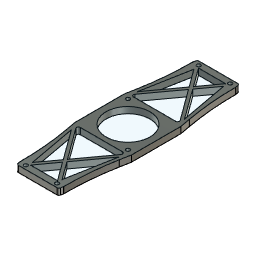
stepper_holding_bracket_printer v3 (Autodesk Fusion 360 design; units mm, degrees)
Autodesk Fusion 360 part; units mm, degrees
note: some values were not read from the file. Set by a fixed rule: which face or edge a step refers to.
sketch "Sketch1" plane through (0, 0, 0) normal (0, 0, 1) x (1, 0, 0)
  line L0 (-21.15, 21.15) -> (21.15, -21.15) construction
  line L1 (21.15, -21.15) -> (-21.15, -21.15)
  line L2 (-21.15, 21.15) -> (-19.0287, 19.0287) construction
  circle A0 centre (0, 0) radius 11
  line L3 (19.0287, 19.0287) -> (21.15, 16.9074)
  line L4 (21.15, 21.15) -> (19.0287, 19.0287) construction
  line L5 (-19.0287, -19.0287) -> (-16.9074, -21.15)
  line L6 (-19.0287, -19.0287) -> (-15.4931, -15.4931) construction
  line L7 (19.0287, 19.0287) -> (16.9074, 21.15)
  line L8 (-19.0287, 19.0287) -> (-21.15, 16.9074)
  line L9 (-19.0287, 19.0287) -> (-16.9074, 21.15)
  line L10 (-21.15, -21.15) -> (-21.15, 21.15)
  line L11 (19.0287, -19.0287) -> (16.9074, -21.15)
  line L12 (-19.0287, 19.0287) -> (-15.4931, 15.4931) construction
  line L13 (-19.0287, -19.0287) -> (-21.15, -16.9074)
  line L14 (21.15, 21.15) -> (-21.15, -21.15) construction
  line L15 (-21.15, -21.15) -> (-19.0287, -19.0287) construction
  line L16 (19.0287, -19.0287) -> (15.4931, -15.4931) construction
  line L17 (21.15, -21.15) -> (19.0287, -19.0287) construction
  line L18 (19.0287, -19.0287) -> (21.15, -16.9074)
  line L19 (19.0287, 19.0287) -> (15.4931, 15.4931) construction
  line L20 (21.15, 21.15) -> (21.15, -21.15)
  line L21 (-21.15, 21.15) -> (21.15, 21.15)
  circle A1 centre (0, 0) radius 2.5
  line L22 (22.5, 75) -> (-14.9629, 75)
  line L23 (-22.5, 75) -> (-22.5, -75)
  line L24 (-22.5, -75) -> (22.5, -75)
  line L25 (22.5, -75) -> (22.5, 75)
  line L26 (22.5, 75) -> (-22.5, -75) construction
  line L27 (-22.5, 75) -> (22.5, -75) construction
  line L28 (-22.5, 69) -> (22.5, 69) construction
  circle A2 centre (-12.5, 69) radius 1.5
  line L29 (-22.5, 0) -> (22.5, 0) construction
  line L30 (0, 75) -> (0, -75) construction
  circle A3 centre (12.5, 69) radius 1.5
  line L31 (-15.7993, 67) -> (22.5, 67)
  line L32 (-12.5559, 67.501) -> (-21.15, 21.15)
  line L33 (-22.5, 19.721) -> (-13.5598, 67.9385)
  line L34 (-21.15, 21.15) -> (-19.8211, 21.15) construction
  line L35 (-19.8211, 21.15) -> (-11.025, 68.7273)
  line L36 (21.15, 21.15) -> (-12.5559, 67.501)
  line L37 (22.5, 21.2586) -> (-11.443, 67.9357)
  line L38 (21.15, 21.15) -> (19.8211, 21.15) construction
  line L39 (-17.2787, 68.7475) -> (-16.4423, 73.7475)
  line L40 (19.8211, 21.15) -> (-13.7338, 67)
  arc A4 (-17.2787, 68.7475) -> (-15.7993, 67) centre (-15.7993, 68.5) ccw
  arc A5 (-14.9629, 75) -> (-16.4423, 73.7475) centre (-14.9629, 73.5) ccw
  line L41 (22.5, 19.721) -> (13.5598, 67.9385)
  line L42 (19.8211, 21.15) -> (11.025, 68.7273)
  line L43 (-19.8211, 21.15) -> (13.7338, 67)
  line L44 (-22.5, 21.2586) -> (11.443, 67.9357)
  arc A6 (15.7993, 67) -> (17.2787, 68.7475) centre (15.7993, 68.5) ccw
  line L45 (17.2787, 68.7475) -> (16.4423, 73.7475)
  arc A7 (16.4423, 73.7475) -> (14.9629, 75) centre (14.9629, 73.5) ccw
  line L46 (-22.5, -19.721) -> (-13.5598, -67.9385)
  line L47 (-19.8211, -21.15) -> (-11.025, -68.7273)
  line L48 (19.8211, -21.15) -> (-13.7338, -67)
  line L49 (22.5, -21.2586) -> (-11.443, -67.9357)
  line L50 (-22.5, -21.2586) -> (11.443, -67.9357)
  line L51 (-19.8211, -21.15) -> (13.7338, -67)
  line L52 (19.8211, -21.15) -> (11.025, -68.7273)
  line L53 (22.5, -19.721) -> (13.5598, -67.9385)
  circle A8 centre (12.5, -69) radius 1.5
  circle A9 centre (-12.5, -69) radius 1.5
  arc A10 (-15.7993, -67) -> (-17.2787, -68.7475) centre (-15.7993, -68.5) ccw
  line L54 (-17.2787, -68.7475) -> (-16.4423, -73.7475)
  arc A11 (-16.4423, -73.7475) -> (-14.9629, -75) centre (-14.9629, -73.5) ccw
  arc A12 (14.9629, -75) -> (16.4423, -73.7475) centre (14.9629, -73.5) ccw
  line L55 (17.2787, -68.7475) -> (16.4423, -73.7475)
  arc A13 (17.2787, -68.7475) -> (15.7993, -67) centre (15.7993, -68.5) ccw
  line L56 (-15.7993, -67) -> (22.5, -67)
  line L57 (0, 0) -> (-17.5716, 17.5716) construction
  line L58 (0, 0) -> (17.5716, -17.5716) construction
  circle A14 centre (17.5716, -17.5716) radius 1.5
  circle A15 centre (-17.5716, 17.5716) radius 1.5
  dimension "d1" = 42.3
  dimension "d2" = 42.3
  dimension "d3" = 3
  dimension "d4" = 3
  dimension "d5" = 3
  dimension "d6" = 3
  dimension "d15" = 5
  dimension "d16" = 22
  dimension "d17" = 45
  dimension "d18" = 150
  dimension "d19" = 6
  dimension "d20" = 3
  dimension "d21" = 10
  dimension "d22" = 8
  dimension "d23" = 1.3289
  dimension "d24" = 1.3289
  dimension "d25" = 1.5
  dimension "d26" = 1.5
  dimension "d50" = 24.85
  dimension "d51" = 24.85
  dimension "d52" = 3
  dimension "d53" = 3
  constraint horizontal L21
  constraint vertical L20
  constraint horizontal L1
  constraint vertical L10
  constraint coincident L5.start L14
  constraint perpendicular L2 L15
  constraint coincident L3.start L14
  constraint coincident L11.start L0
  constraint coincident L11.end L1
  constraint perpendicular L0 L11
  constraint coincident L18.end L20
  constraint perpendicular L0 L18
  constraint coincident L5.end L1
  constraint perpendicular L5 L15
  constraint coincident L13.end L10
  constraint perpendicular L13 L14
  constraint coincident L8.end L10
  constraint perpendicular L0 L8
  constraint coincident L9.end L21
  constraint perpendicular L0 L9
  constraint coincident L3.end L20
  constraint perpendicular L3 L14
  constraint coincident L7.end L21
  constraint perpendicular L4 L7
  constraint coincident L19.end L14
  constraint coincident L12.end L0
  constraint coincident L6.end L14
  constraint coincident L16.end L0
  constraint midpoint A0.centre L0
  constraint concentric A0 A1
  constraint horizontal L22
  constraint perpendicular L22 L23
  constraint parallel L22 L24
  constraint parallel L23 L25
  constraint coincident L26 A0.centre
  constraint coincident L27 A0.centre
  constraint coincident A0.centre A1.centre
  constraint coincident L23 L28.start
  constraint coincident L25 L28.end
  constraint perpendicular L25 L28
  constraint coincident L28 A2.centre
  constraint midpoint L23 L29.start
  constraint midpoint L25 L29.end
  constraint midpoint L24 L30.end
  constraint symmetric A2 L30 A3
  constraint coincident L25 L31.end
  constraint perpendicular L25 L31
  constraint coincident A2 L32.start
  constraint coincident L23 L33.start
  constraint coincident A2 L33.end
  constraint parallel L32 L33
  constraint coincident L21 L34.end
  constraint coincident A2 L35.end
  constraint tangent A2 L35
  constraint coincident L25 L37.start
  constraint coincident A2 L37.end
  constraint parallel L36 L37
  constraint coincident L21 L38.end
  constraint coincident L33 L40.end
  constraint tangent L39 A4
  constraint tangent L31 A4
  constraint coincident L22 L30.start
  constraint coincident L23.start L22
  constraint tangent L39 A5
  constraint tangent L22 A5
  constraint symmetric L30 L33.start L41.start
  constraint symmetric L30 L33.end L41.end
  constraint symmetric L30 L34.end L38.end
  constraint symmetric L30 L35.end L42.end
  constraint symmetric L30 L37.start L44.start
  constraint symmetric L30 L37.end L44.end
  constraint symmetric L30 L38.end L34.end
  constraint symmetric L30 L40.end L43.end
  constraint symmetric L30 L39.start A6.end
  constraint symmetric L30 L31.start A6.start
  constraint symmetric L30 A4 A6
  constraint symmetric L30 L39.end L45.end
  constraint symmetric L30 L22.end A7.end
  constraint symmetric L30 A5 A7
  constraint symmetric A2 L29 A9
  constraint symmetric L29 A3 A8
  constraint symmetric L29 L31.end L56.end
  constraint symmetric L29 L33.start L46.start
  constraint symmetric L29 L33.end L46.end
  constraint symmetric L29 L34.end L47.start
  constraint symmetric L29 L35.end L47.end
  constraint symmetric L29 L37.start L49.start
  constraint symmetric L29 L37.end L49.end
  constraint symmetric L29 L38.end L48.start
  constraint symmetric L29 L40.end L48.end
  constraint symmetric L29 L39.start A10.end
  constraint symmetric L29 L31.start A10.start
  constraint symmetric L29 A4 A10
  constraint symmetric L29 L39.end L54.end
  constraint symmetric L29 L22.end A11.end
  constraint symmetric L29 A5 A11
  constraint symmetric L29 L41.start L53.start
  constraint symmetric L29 L41.end L53.end
  constraint symmetric L29 L42.end L52.end
  constraint symmetric L29 L43.end L51.end
  constraint symmetric L29 L44.start L50.start
  constraint symmetric L29 L44.end L50.end
  constraint symmetric L29 A6.end L55.start
  constraint symmetric L29 A6.start A13.end
  constraint symmetric L29 A6 A13
  constraint symmetric L29 L45.end A12.end
  constraint symmetric L29 A7.end A12.start
  constraint symmetric L29 A7 A12
  constraint coincident L31 L40.end
  constraint parallel L0 L57
  constraint coincident L16 L58.end
  constraint coincident L58.end A14.centre
  constraint coincident L57.end A15.centre
  measures "d1" distance of L1.end L0.start
  measures "d2" distance of L0.start L4.start
  measures "d3" distance of L1.end L5.start
  measures "d4" distance of L0.start L2.end
  measures "d5" distance of L4.start L3.start
  measures "d6" distance of L11.start L0.end
  measures "d15" diameter of A1
  measures "d16" diameter of A0
  measures "d17" distance of L23.end L24.end
  measures "d18" distance of L23.start L23.end
  measures "d19" distance of L22 L28
  measures "d20" diameter of A2
  measures "d21" distance of L23 A2.centre
  measures "d22" distance of L22 L31
  measures "d23" distance of L0.start L34.end
  measures "d24" distance of L4.start L38.end
  measures "d25" radius of A4
  measures "d26" radius of A5
  measures "d50" distance of A0.centre L57.end
  measures "d51" distance of A0.centre L58.end
  measures "d52" diameter of A14
  measures "d53" diameter of A15
extrude "Extrude1" add sketch "Sketch1" along normal blind 5 contours L1 L20 L25 L36 L37 L41 L42 L49 L52 L53 | L1 L11 L18 L20 | L48 L49 L51 L52 | L1 L3 L5 L7 L8 L9 L10 L11 L13 L18 L20 L21 | L48 L49 L50 L51 | L47 L48 L50 L51 | L49 L51 L52 L53 | L3 L7 L20 L21 | L1 L5 L10 L13 | L47 L48 L49 L50 L56 | L1 L10 L23 L32 L33 L44 L46 L47 L50 | L49 L50 L51 L52 L56 | L51 L52 L56 | L21 L36 L42 | L46 L47 L48 L50 | L47 L48 L56 | L24 L46 L47 L49 L50 L52 L53 A8 A9 A10 L54 A11 A12 L55 A13 L56 | L50 L52 L53 A8 L56 | L50 L52 L56 | L36 L40 L42 L43 | L36 L37 L42 L43 | L47 L49 L56 | L46 L47 L49 A9 L56 | L50 L52 A8 | L8 L9 L10 L21 | L35 L40 L43 L44 | L36 L40 L43 L44 | L36 L37 L43 L44 | L37 L41 L42 L43 | L47 L49 A9 | L21 L32 L35 L44 | L35 L36 L40 L44 | L31 L35 L36 L37 L44 | L31 L37 L42 L43 L44 | L31 L42 L43 | L22 A2 A3 L31 L33 L35 L37 L39 A4 A5 L41 L42 L44 A6 L45 A7 | A3 L31 L41 L42 L44 | L32 L35 L40 L44 | L31 L32 L35 L36 L40 | L31 L35 L36 | L31 L42 L44 | L32 L33 L40 L44 | L31 L32 L40 | L31 L35 L37 | A2 L31 L35 L36 L37 | L31 L32 L36 | A3 L42 L44 | A2 L31 L32 L33 | A2 L35 L37 | A14 | A15
fillet "Fillet1" radius 1.5 4 edges at (19.8211, 21.15, 2.5) (-19.8211, 21.15, 2.5) (19.8211, -21.15, 2.5) (-19.8211, -21.15, 2.5)
fillet "Fillet2" radius 219.5 4 edges at (-13.7338, 67, 2.5) (13.7338, 67, 2.5) (-13.7338, -67, 2.5) (13.7338, -67, 2.5)
sketch "Sketch2" plane through (0, 0, 5) normal (0, 0, 1) x (-1, 0, 0)
  line L0 (-11.8262, -64.3935) -> (-18.8809, -26.2354)
  line L1 (-18.8809, -26.2354) -> (-1.4466, -50.2105)
  line L2 (-1.4466, -50.2105) -> (-11.8262, -64.3935)
  circle A0 centre (-12.5, -69) radius 1.5
  line L3 (18.8809, 26.2354) -> (1.4466, 50.2105)
  line L4 (1.4466, 50.2105) -> (11.8262, 64.3935)
  line L5 (11.8262, 64.3935) -> (18.8809, 26.2354)
  line L6 (10.7626, 67) -> (0, 52.1997)
  line L7 (0, 52.1997) -> (-10.7626, 67)
  line L8 (-10.7626, 67) -> (10.7626, 67)
  circle A1 centre (12.5, 69) radius 1.5
  circle A2 centre (-12.5, 69) radius 1.5
  line L9 (0, -48.2339) -> (-18.075, -23.5359)
  arc A3 (-16.8646, -21.15) -> (-18.075, -23.5359) centre (-16.8646, -22.65) ccw
  line L10 (-16.8646, -21.15) -> (16.8646, -21.15)
  arc A4 (18.075, -23.5359) -> (16.8646, -21.15) centre (16.8646, -22.65) ccw
  line L11 (18.075, -23.5359) -> (0, -48.2339)
  circle A5 centre (12.5, -69) radius 1.5
  line L12 (16.8646, 21.15) -> (-16.8646, 21.15)
  arc A6 (-18.075, 23.5359) -> (-16.8646, 21.15) centre (-16.8646, 22.65) ccw
  line L13 (-18.075, 23.5359) -> (0, 48.2339)
  line L14 (0, 48.2339) -> (18.075, 23.5359)
  arc A7 (16.8646, 21.15) -> (18.075, 23.5359) centre (16.8646, 22.65) ccw
  line L15 (-10.7626, -67) -> (0, -52.1997)
  line L16 (0, -52.1997) -> (10.7626, -67)
  line L17 (10.7626, -67) -> (-10.7626, -67)
  line L18 (11.8262, -64.3935) -> (1.4466, -50.2105)
  line L19 (1.4466, -50.2105) -> (18.8809, -26.2354)
  line L20 (18.8809, -26.2354) -> (11.8262, -64.3935)
  circle A8 centre (0, 0) radius 11
  line L21 (-1.4466, 50.2105) -> (-18.8809, 26.2354)
  line L22 (-18.8809, 26.2354) -> (-11.8262, 64.3935)
  line L23 (-11.8262, 64.3935) -> (-1.4466, 50.2105)
  line L24 (17.2787, 68.7475) -> (16.4423, 73.7475)
  arc A9 (16.4423, 73.7475) -> (14.9629, 75) centre (14.9629, 73.5) ccw
  line L25 (14.9629, 75) -> (-14.9629, 75)
  arc A10 (-14.9629, 75) -> (-16.4423, 73.7475) centre (-14.9629, 73.5) ccw
  line L26 (-16.4423, 73.7475) -> (-17.2787, 68.7475)
  arc A11 (-17.2787, 68.7475) -> (-17.2992, 68.4963) centre (-15.7993, 68.5) ccw
  arc A12 (-20.977, 27.9349) -> (-17.2992, 68.4963) centre (-236.7986, 67.9512) ccw
  line L27 (-20.977, 27.9349) -> (-22.5, 19.721)
  line L28 (-22.5, 19.721) -> (-22.5, -19.721)
  line L29 (-22.5, -19.721) -> (-20.977, -27.9349)
  arc A13 (-17.2992, -68.4963) -> (-20.977, -27.9349) centre (-236.7986, -67.9512) ccw
  arc A14 (-17.2992, -68.4963) -> (-17.2787, -68.7475) centre (-15.7993, -68.5) ccw
  line L30 (-17.2787, -68.7475) -> (-16.4423, -73.7475)
  arc A15 (-16.4423, -73.7475) -> (-14.9629, -75) centre (-14.9629, -73.5) ccw
  line L31 (-14.9629, -75) -> (14.9629, -75)
  arc A16 (14.9629, -75) -> (16.4423, -73.7475) centre (14.9629, -73.5) ccw
  line L32 (16.4423, -73.7475) -> (17.2787, -68.7475)
  arc A17 (17.2787, -68.7475) -> (17.2992, -68.4963) centre (15.7993, -68.5) ccw
  arc A18 (20.977, -27.9349) -> (17.2992, -68.4963) centre (236.7986, -67.9512) ccw
  line L33 (20.977, -27.9349) -> (22.5, -19.721)
  line L34 (22.5, -19.721) -> (22.5, 19.721)
  line L35 (22.5, 19.721) -> (20.977, 27.9349)
  arc A19 (17.2992, 68.4963) -> (20.977, 27.9349) centre (236.7986, 67.9512) ccw
  arc A20 (17.2992, 68.4963) -> (17.2787, 68.7475) centre (15.7993, 68.5) ccw
  circle A21 centre (-15.4931, 15.4931) radius 3.5
  line L36 (-22.5, 0) -> (22.5, 0) construction
  line L37 (0, 0) -> (0, 75) construction
  circle A22 centre (15.4931, 15.4931) radius 3.5
  line L38 (-15.4931, 15.4931) -> (-11.9931, 15.4931) construction
  circle A23 centre (0, 142.5886) radius 124.5363 construction
  circle A24 centre (0, 142.5886) radius 131.5363 construction
  circle A25 centre (0, 0) radius 13.5
  arc A26 (-13.268, 2.4919) -> (-17.4643, 12.601) centre (-23.0962, 4.3377) ccw
  arc A27 (-12.601, 17.4643) -> (-2.4919, 13.268) centre (-4.3377, 23.0962) ccw
  arc A28 (17.4643, 12.601) -> (13.268, 2.4919) centre (23.0962, 4.3377) ccw
  arc A29 (2.4919, 13.268) -> (12.601, 17.4643) centre (4.3377, 23.0962) ccw
  arc A30 (-17.4643, -12.601) -> (-13.268, -2.4919) centre (-23.0962, -4.3377) ccw
  arc A31 (-2.4919, -13.268) -> (-12.601, -17.4643) centre (-4.3377, -23.0962) ccw
  circle A32 centre (-15.4931, -15.4931) radius 3.5
  arc A33 (12.601, -17.4643) -> (2.4919, -13.268) centre (4.3377, -23.0962) ccw
  arc A34 (13.268, -2.4919) -> (17.4643, -12.601) centre (23.0962, -4.3377) ccw
  circle A35 centre (15.4931, -15.4931) radius 3.5
  line L39 (-15.4931, 15.4931) -> (-15.4931, 18.9931) construction
  line L40 (-15.4931, 18.9931) -> (15.4931, 18.9931)
  line L41 (-18.9931, 15.4931) -> (-18.9931, -15.4931)
  line L42 (-15.4931, -18.9931) -> (15.4931, -18.9931)
  line L43 (18.9931, -15.4931) -> (18.9931, 15.4931)
  line L44 (13.105, 4.7569) -> (13.105, -4.7569)
  line L45 (-13.105, 4.7569) -> (-13.105, -4.7569)
  line L46 (4.7605, -0.0581) -> (-4.7533, -0.0581)
  line L47 (0, 0) -> (0, -13.105) construction
  line L48 (0, -13.105) -> (4.3174, -13.0962) construction
  line L49 (4.3174, -13.0962) -> (-4.3377, -13.0962)
  line L50 (4.3174, 13.0962) -> (-4.3377, 13.0962)
  arc A36 (16.9784, -12.248) -> (18.9931, -11.2592) centre (17.7431, -11.2592) ccw
  arc A37 (11.2592, -18.9931) -> (12.248, -16.9784) centre (11.2592, -17.7431) ccw
  arc A38 (-12.248, -16.9784) -> (-11.2592, -18.9931) centre (-11.2592, -17.7431) ccw
  arc A39 (-18.9931, -11.2592) -> (-16.9784, -12.248) centre (-17.7431, -11.2592) ccw
  arc A40 (18.9931, 11.2592) -> (16.9784, 12.248) centre (17.7431, 11.2592) ccw
  arc A41 (12.248, 16.9784) -> (11.2592, 18.9931) centre (11.2592, 17.7431) ccw
  arc A42 (-11.2592, 18.9931) -> (-12.248, 16.9784) centre (-11.2592, 17.7431) ccw
  arc A43 (-16.9784, 12.248) -> (-18.9931, 11.2592) centre (-17.7431, 11.2592) ccw
  dimension "d33" = 7
  dimension "d36" = 7
  dimension "d37" = 27
  dimension "d38" = 20
  dimension "d39" = 20
  dimension "d40" = 13.105
  dimension "d43" = 2.5
  dimension "d44" = 2.5
  constraint midpoint L28 L36.start
  constraint midpoint L34 L36.end
  constraint coincident A8.centre L37.start
  constraint midpoint L25 L37.end
  constraint symmetric A21 L37 A22
  constraint horizontal L38
  constraint tangent A21 A23
  constraint tangent A22 A23
  constraint tangent A21 A26
  constraint tangent A25 A26
  constraint tangent A25 A27
  constraint tangent A21 A27
  constraint coincident A25 A26.start
  constraint coincident A21 A26.end
  constraint coincident A25 A27.end
  constraint coincident A21 A27.start
  constraint symmetric L37 A26.start A28.end
  constraint symmetric L37 A26.end A28.start
  constraint symmetric L37 A26 A28
  constraint symmetric L37 A27.end A29.start
  constraint symmetric L37 A27 A29
  constraint symmetric L37 A27.start A29.end
  constraint symmetric A21 L36 A32
  constraint symmetric L36 A22 A35
  constraint symmetric L36 A26.start A30.end
  constraint symmetric L36 A26.end A30.start
  constraint symmetric L36 A26 A30
  constraint symmetric L36 A27.end A31.start
  constraint symmetric L36 A27 A31
  constraint symmetric L36 A27.start A31.end
  constraint symmetric L36 A28.end A34.start
  constraint symmetric L36 A28.start A34.end
  constraint symmetric L36 A28 A34
  constraint symmetric L36 A29.end A33.start
  constraint symmetric L36 A29.start A33.end
  constraint symmetric L36 A29 A33
  constraint coincident A21 L39.end
  constraint perpendicular L38 L39
  constraint coincident A22 L40.end
  constraint tangent A22 L40
  constraint coincident A21 L41.start
  constraint coincident A32 L41.end
  constraint tangent A32 L41
  constraint perpendicular L36 L41
  constraint coincident A32 L42.start
  constraint coincident A35 L42.end
  constraint tangent A35 L42
  constraint perpendicular L41 L42
  constraint coincident A35 L43.start
  constraint coincident A22 L43.end
  constraint tangent A22 L43
  constraint perpendicular L42 L43
  constraint coincident A28 L44.start
  constraint coincident A34 L44.end
  constraint perpendicular L36 L44
  constraint symmetric L37 L44.start L45.start
  constraint symmetric L37 L44.end L45.end
  constraint perpendicular L46 L47
  constraint coincident A33 L48.end
  constraint tangent A33 L48
  constraint coincident A31 L49.end
  constraint tangent A31 L49
  constraint symmetric L36 L48.end L50.start
  constraint symmetric L36 L49.end L50.end
  constraint tangent L43 A36
  constraint tangent A34 A36
  constraint tangent L42 A37
  constraint tangent A33 A37
  constraint coincident L43 A36.end
  constraint coincident A34 A36.start
  constraint coincident A33 A37.end
  constraint coincident L42 A37.start
  constraint symmetric L47 A36.end A39.start
  constraint symmetric L47 A36.start A39.end
  constraint symmetric L47 A36 A39
  constraint symmetric L47 A37.end A38.start
  constraint symmetric L47 A37.start A38.end
  constraint symmetric L47 A37 A38
  constraint symmetric L36 A36.end A40.start
  constraint symmetric L36 A36.start A40.end
  constraint symmetric L36 A36 A40
  constraint symmetric L36 A37.end A41.start
  constraint symmetric L36 A37.start A41.end
  constraint symmetric L36 A37 A41
  constraint symmetric L36 A38.end A42.start
  constraint symmetric L36 A38.start A42.end
  constraint symmetric L36 A38 A42
  constraint symmetric L36 A39.end A43.start
  constraint symmetric L36 A39.start A43.end
  constraint symmetric L36 A39 A43
  measures "d33" diameter of A21
  measures "d37" diameter of A25
  measures "d38" diameter of A26
  measures "d39" diameter of A27
  measures "d40" distance of A8.centre L47.end
  measures "d43" diameter of A36
  measures "d44" diameter of A37
extrude "Extrude2" [suppressed]
sketch "Sketch3" plane through (0, 0, 5) normal (0, 0, 1) x (-1, 0, 0)
  line L0 (-11.8262, -64.3935) -> (-18.8809, -26.2354)
  line L1 (-18.8809, -26.2354) -> (-1.4466, -50.2105)
  line L2 (-1.4466, -50.2105) -> (-11.8262, -64.3935)
  circle A0 centre (-12.5, -69) radius 1.5
  line L3 (18.8809, 26.2354) -> (1.4466, 50.2105)
  line L4 (1.4466, 50.2105) -> (11.8262, 64.3935)
  line L5 (11.8262, 64.3935) -> (18.8809, 26.2354)
  line L6 (10.7626, 67) -> (0, 52.1997)
  line L7 (0, 52.1997) -> (-10.7626, 67)
  line L8 (-10.7626, 67) -> (10.7626, 67)
  circle A1 centre (12.5, 69) radius 1.5
  circle A2 centre (-12.5, 69) radius 1.5
  line L9 (0, -48.2339) -> (-18.075, -23.5359)
  arc A3 (-16.8646, -21.15) -> (-18.075, -23.5359) centre (-16.8646, -22.65) ccw
  line L10 (-16.8646, -21.15) -> (16.8646, -21.15)
  arc A4 (18.075, -23.5359) -> (16.8646, -21.15) centre (16.8646, -22.65) ccw
  line L11 (18.075, -23.5359) -> (0, -48.2339)
  circle A5 centre (12.5, -69) radius 1.5
  line L12 (16.8646, 21.15) -> (-16.8646, 21.15)
  arc A6 (-18.075, 23.5359) -> (-16.8646, 21.15) centre (-16.8646, 22.65) ccw
  line L13 (-18.075, 23.5359) -> (0, 48.2339)
  line L14 (0, 48.2339) -> (18.075, 23.5359)
  arc A7 (16.8646, 21.15) -> (18.075, 23.5359) centre (16.8646, 22.65) ccw
  line L15 (-10.7626, -67) -> (0, -52.1997)
  line L16 (0, -52.1997) -> (10.7626, -67)
  line L17 (10.7626, -67) -> (-10.7626, -67)
  line L18 (11.8262, -64.3935) -> (1.4466, -50.2105)
  line L19 (1.4466, -50.2105) -> (18.8809, -26.2354)
  line L20 (18.8809, -26.2354) -> (11.8262, -64.3935)
  circle A8 centre (0, 0) radius 11
  line L21 (-1.4466, 50.2105) -> (-18.8809, 26.2354)
  line L22 (-18.8809, 26.2354) -> (-11.8262, 64.3935)
  line L23 (-11.8262, 64.3935) -> (-1.4466, 50.2105)
  line L24 (17.2787, 68.7475) -> (16.4423, 73.7475)
  arc A9 (16.4423, 73.7475) -> (14.9629, 75) centre (14.9629, 73.5) ccw
  line L25 (14.9629, 75) -> (-14.9629, 75)
  arc A10 (-14.9629, 75) -> (-16.4423, 73.7475) centre (-14.9629, 73.5) ccw
  line L26 (-16.4423, 73.7475) -> (-17.2787, 68.7475)
  arc A11 (-17.2787, 68.7475) -> (-17.2992, 68.4963) centre (-15.7993, 68.5) ccw
  arc A12 (-20.977, 27.9349) -> (-17.2992, 68.4963) centre (-236.7986, 67.9512) ccw
  line L27 (-20.977, 27.9349) -> (-22.5, 19.721)
  line L28 (-22.5, 19.721) -> (-22.5, -19.721)
  line L29 (-22.5, -19.721) -> (-20.977, -27.9349)
  arc A13 (-17.2992, -68.4963) -> (-20.977, -27.9349) centre (-236.7986, -67.9512) ccw
  arc A14 (-17.2992, -68.4963) -> (-17.2787, -68.7475) centre (-15.7993, -68.5) ccw
  line L30 (-17.2787, -68.7475) -> (-16.4423, -73.7475)
  arc A15 (-16.4423, -73.7475) -> (-14.9629, -75) centre (-14.9629, -73.5) ccw
  line L31 (-14.9629, -75) -> (14.9629, -75)
  arc A16 (14.9629, -75) -> (16.4423, -73.7475) centre (14.9629, -73.5) ccw
  line L32 (16.4423, -73.7475) -> (17.2787, -68.7475)
  arc A17 (17.2787, -68.7475) -> (17.2992, -68.4963) centre (15.7993, -68.5) ccw
  arc A18 (20.977, -27.9349) -> (17.2992, -68.4963) centre (236.7986, -67.9512) ccw
  line L33 (20.977, -27.9349) -> (22.5, -19.721)
  line L34 (22.5, -19.721) -> (22.5, 19.721)
  line L35 (22.5, 19.721) -> (20.977, 27.9349)
  arc A19 (17.2992, 68.4963) -> (20.977, 27.9349) centre (236.7986, 67.9512) ccw
  arc A20 (17.2992, 68.4963) -> (17.2787, 68.7475) centre (15.7993, 68.5) ccw
  circle A21 centre (0, 0) radius 17.5
  dimension "d45" = 35
  constraint coincident A8.centre A21.centre
  measures "d45" diameter of A21
extrude "Extrude3" cut sketch "Sketch3" against normal blind 5 contours A21
move_face "OffsetFaces1" offset -3 1 faces at (-4.9876, -75, 3.3333)
move_face "OffsetFaces2" offset -3 1 faces at (4.9876, 75, 1.6667)
sketch "Sketch4" plane through (0, 0, 0) normal (0, 0, 1) x (1, 0, 0)
extrude "Extrude4" cut sketch "Sketch1" along normal blind 5 contours A14 | A15
sketch "Sketch5" plane through (0, 0, 5) normal (0, 0, 1) x (-1, 0, 0)
  circle A0 centre (-17.5716, 17.5716) radius 1.5
  circle A1 centre (17.5716, -17.5716) radius 1.5
  arc A2 (-16.9441, -70.7475) -> (-15.4647, -72) centre (-15.4647, -70.5) ccw
  line L0 (-15.4647, -72) -> (15.4647, -72)
  arc A3 (15.4647, -72) -> (16.9441, -70.7475) centre (15.4647, -70.5) ccw
  line L1 (16.9441, -70.7475) -> (17.2787, -68.7475)
  arc A4 (17.2787, -68.7475) -> (17.2992, -68.4963) centre (15.7993, -68.5) ccw
  arc A5 (20.977, -27.9349) -> (17.2992, -68.4963) centre (236.7986, -67.9512) ccw
  line L2 (20.977, -27.9349) -> (22.5, -19.721)
  line L3 (22.5, -19.721) -> (22.5, 19.721)
  line L4 (22.5, 19.721) -> (20.977, 27.9349)
  arc A6 (17.2992, 68.4963) -> (20.977, 27.9349) centre (236.7986, 67.9512) ccw
  arc A7 (17.2992, 68.4963) -> (17.2787, 68.7475) centre (15.7993, 68.5) ccw
  line L5 (17.2787, 68.7475) -> (16.9441, 70.7475)
  arc A8 (16.9441, 70.7475) -> (15.4647, 72) centre (15.4647, 70.5) ccw
  line L6 (15.4647, 72) -> (-15.4647, 72)
  arc A9 (-15.4647, 72) -> (-16.9441, 70.7475) centre (-15.4647, 70.5) ccw
  line L7 (-16.9441, 70.7475) -> (-17.2787, 68.7475)
  arc A10 (-17.2787, 68.7475) -> (-17.2992, 68.4963) centre (-15.7993, 68.5) ccw
  arc A11 (-20.977, 27.9349) -> (-17.2992, 68.4963) centre (-236.7986, 67.9512) ccw
  line L8 (-20.977, 27.9349) -> (-22.5, 19.721)
  line L9 (-22.5, 19.721) -> (-22.5, -19.721)
  line L10 (-22.5, -19.721) -> (-20.977, -27.9349)
  arc A12 (-17.2992, -68.4963) -> (-20.977, -27.9349) centre (-236.7986, -67.9512) ccw
  arc A13 (-17.2992, -68.4963) -> (-17.2787, -68.7475) centre (-15.7993, -68.5) ccw
  line L11 (-17.2787, -68.7475) -> (-16.9441, -70.7475)
  circle A14 centre (0, 0) radius 17.5
  line L12 (11.8262, -64.3935) -> (1.4466, -50.2105)
  line L13 (1.4466, -50.2105) -> (18.8809, -26.2354)
  line L14 (18.8809, -26.2354) -> (11.8262, -64.3935)
  circle A15 centre (12.5, -69) radius 1.5
  circle A16 centre (-12.5, 69) radius 1.5
  circle A17 centre (-12.5, -69) radius 1.5
  line L15 (0, -48.2339) -> (-18.075, -23.5359)
  arc A18 (-16.8646, -21.15) -> (-18.075, -23.5359) centre (-16.8646, -22.65) ccw
  line L16 (-16.8646, -21.15) -> (16.8646, -21.15)
  arc A19 (18.075, -23.5359) -> (16.8646, -21.15) centre (16.8646, -22.65) ccw
  line L17 (18.075, -23.5359) -> (0, -48.2339)
  line L18 (-11.8262, -64.3935) -> (-18.8809, -26.2354)
  line L19 (-18.8809, -26.2354) -> (-1.4466, -50.2105)
  line L20 (-1.4466, -50.2105) -> (-11.8262, -64.3935)
  line L21 (16.8646, 21.15) -> (-16.8646, 21.15)
  arc A20 (-18.075, 23.5359) -> (-16.8646, 21.15) centre (-16.8646, 22.65) ccw
  line L22 (-18.075, 23.5359) -> (0, 48.2339)
  line L23 (0, 48.2339) -> (18.075, 23.5359)
  arc A21 (16.8646, 21.15) -> (18.075, 23.5359) centre (16.8646, 22.65) ccw
  line L24 (-10.7626, -67) -> (0, -52.1997)
  line L25 (0, -52.1997) -> (10.7626, -67)
  line L26 (10.7626, -67) -> (-10.7626, -67)
  circle A22 centre (12.5, 69) radius 1.5
  line L27 (10.7626, 67) -> (0, 52.1997)
  line L28 (0, 52.1997) -> (-10.7626, 67)
  line L29 (-10.7626, 67) -> (10.7626, 67)
  line L30 (18.8809, 26.2354) -> (1.4466, 50.2105)
  line L31 (1.4466, 50.2105) -> (11.8262, 64.3935)
  line L32 (11.8262, 64.3935) -> (18.8809, 26.2354)
  line L33 (-1.4466, 50.2105) -> (-18.8809, 26.2354)
  line L34 (-18.8809, 26.2354) -> (-11.8262, 64.3935)
  line L35 (-11.8262, 64.3935) -> (-1.4466, 50.2105)
named bodies: "stepper_holding_bracket"
